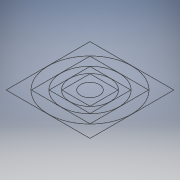
# Autodesk Inventor part: bed leveling
Saved by Autodesk Inventor 2019.3 (Build 233278000, 278)
## iProperties
Created: 2019-06-05
Part Number: bed leveling
Material: Generic
Document SubType Name: Modeling
Designer: Frienddo
Density: 1 g/cm^3
Appearance: Default
Author: Frienddo
Autodesk Inventor part; units mm, degrees
ref_plane "YZ Plane" through (0, 0, 0) normal (1, 0, 0) x (0, 1, 0)
ref_plane "XZ Plane" through (0, 0, 0) normal (0, 1, 0) x (-1, 0, 0)
ref_plane "XY Plane" through (0, 0, 0) normal (0, 0, 1) x (1, 0, 0)
sketch "Sketch1" plane through (0, 0, 0) normal (0, 1, 0) x (-1, 0, 0)
  line L0 (-135, -135) -> (135, -135)
  line L1 (135, -135) -> (135, 135)
  line L2 (135, 135) -> (-135, 135)
  line L3 (-135, 135) -> (-135, -135)
  line L4 (-135, -135) -> (135, 135) construction
  line L5 (135, -135) -> (-135, 135) construction
  line L6 (134.3, 134.3) -> (134.3, -134.3)
  line L7 (134.3, -134.3) -> (-134.3, -134.3)
  line L8 (-134.3, -134.3) -> (-134.3, 134.3)
  line L9 (-134.3, 134.3) -> (134.3, 134.3)
  circle A0 centre (0, 0) radius 134.3
  circle A1 centre (0, 0) radius 133.6
  line L10 (-94.4695, -94.4695) -> (94.4695, -94.4695)
  line L11 (94.4695, -94.4695) -> (94.4695, 94.4695)
  line L12 (94.4695, 94.4695) -> (-94.4695, 94.4695)
  line L13 (-94.4695, 94.4695) -> (-94.4695, -94.4695)
  line L14 (-94.4695, -94.4695) -> (94.4695, 94.4695) construction
  line L15 (94.4695, -94.4695) -> (-94.4695, 94.4695) construction
  line L16 (93.7695, 93.7695) -> (93.7695, -93.7695)
  line L17 (93.7695, -93.7695) -> (-93.7695, -93.7695)
  line L18 (-93.7695, -93.7695) -> (-93.7695, 93.7695)
  line L19 (-93.7695, 93.7695) -> (93.7695, 93.7695)
  circle A2 centre (0, 0) radius 93.7695
  circle A3 centre (0, 0) radius 93.0695
  line L20 (-65.8101, -65.8101) -> (65.8101, -65.8101)
  line L21 (65.8101, -65.8101) -> (65.8101, 65.8101)
  line L22 (65.8101, 65.8101) -> (-65.8101, 65.8101)
  line L23 (-65.8101, 65.8101) -> (-65.8101, -65.8101)
  line L24 (-65.8101, -65.8101) -> (65.8101, 65.8101) construction
  line L25 (65.8101, -65.8101) -> (-65.8101, 65.8101) construction
  line L26 (65.1101, 65.1101) -> (65.1101, -65.1101)
  line L27 (65.1101, -65.1101) -> (-65.1101, -65.1101)
  line L28 (-65.1101, -65.1101) -> (-65.1101, 65.1101)
  line L29 (-65.1101, 65.1101) -> (65.1101, 65.1101)
  circle A4 centre (0, 0) radius 65.1101
  circle A5 centre (0, 0) radius 64.4101
  line L30 (-45.5448, -45.5448) -> (45.5448, -45.5448)
  line L31 (45.5448, -45.5448) -> (45.5448, 45.5448)
  line L32 (45.5448, 45.5448) -> (-45.5448, 45.5448)
  line L33 (-45.5448, 45.5448) -> (-45.5448, -45.5448)
  line L34 (-45.5448, -45.5448) -> (45.5448, 45.5448) construction
  line L35 (45.5448, -45.5448) -> (-45.5448, 45.5448) construction
  line L36 (44.8448, 44.8448) -> (44.8448, -44.8448)
  line L37 (44.8448, -44.8448) -> (-44.8448, -44.8448)
  line L38 (-44.8448, -44.8448) -> (-44.8448, 44.8448)
  line L39 (-44.8448, 44.8448) -> (44.8448, 44.8448)
  circle A6 centre (0, 0) radius 30
  circle A7 centre (0, 0) radius 30.7
  dimension "d0" = 270
  dimension "d1" = 270
  dimension "d2" = 0.7
  dimension "d3" = 0.7
  dimension "d4" = 0.7
  dimension "d5" = 0.7
  dimension "d6" = 0.7
  dimension "d7" = 0.7
  dimension "d8" = 0.7
  dimension "d9" = 60
  dimension "d10" = 0.7
  constraints: 80 end point, 16 parallel, 8 midpoint, 8 perpendicular, 5 centre point, 4 coincident, 4 horizontal, 3 point on line, 3 tangent, 21 other
  measures "d0" distance of L2.end L1.end
  measures "d1" distance between parallel lines of L0 L2
  measures "d2" distance between parallel lines of L1 L6
  measures "d4" distance between parallel lines of L11 L16
  measures "d6" distance between parallel lines of L21 L26
  measures "d8" distance between parallel lines of L31 L36
  measures "d9" diameter of A6
  measures "d10" radial gap between concentric circles of A6 A7
extrude "Extrusion1" add sketch "Sketch1" along normal blind 0.35 contours L3 L2 L1 L0 | A0 | L11 L10 L13 L12 | A2 | L21 L20 L23 L22 | A4 | L31 L30 L33 L32 | A7
body "Solid1"
